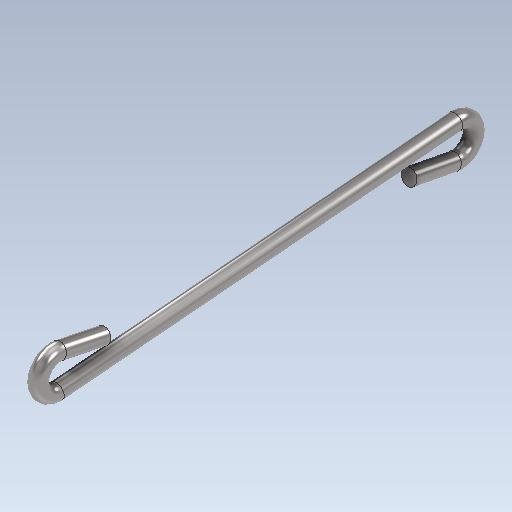
# Autodesk Inventor part: link_4
Saved by Autodesk Inventor 2021 (Build 250183000, 183)
## iProperties
Created: 2023-08-18
Part Number: link_4
Material: Acero inoxidable, 440C
Document SubType Name: Modeling
Designer: Sergio
Density: 7.75 g/cm^3
Appearance: Semipulido
Author: Sergio
Autodesk Inventor part; units mm, degrees
ref_plane "YZ Plane" through (0, 0, 0) normal (1, 0, 0) x (0, 1, 0)
ref_plane "XZ Plane" through (0, 0, 0) normal (0, 1, 0) x (-1, 0, 0)
ref_plane "XY Plane" through (0, 0, 0) normal (0, 0, 1) x (1, 0, 0)
sketch "Boceto1" plane through (0, 0, 0) normal (1, 0, 0) x (0, 1, 0)
  arc A0 (-1.3752, 0.2625) -> (1.3949, 0.119) centre (0, 0) ccw
  line L0 (-1.3949, 59.881) -> (3.6866, 0.3145)
  line L1 (-3.6866, 59.6855) -> (1.3949, 0.119)
  line L2 (-2.5408, 59.7832) -> (2.5408, 0.2168)
  line L3 (0, 53.1) -> (1.3709, 59.7159)
  line L4 (2.2522, 52.6333) -> (3.623, 59.2493)
  line L5 (1.1261, 52.8667) -> (2.497, 59.4826)
  line L6 (-0.1083, 6.8991) -> (-1.3752, 0.2625)
  arc A1 (-2.5048, 0.4781) -> (2.5408, 0.2168) centre (0, 0) ccw
  arc A2 (-3.6344, 0.6937) -> (3.6866, 0.3145) centre (0, 0) ccw
  arc A3 (3.623, 59.2493) -> (-3.6866, 59.6855) centre (0, 60) ccw
  arc A4 (2.497, 59.4826) -> (-2.5408, 59.7832) centre (0, 60) ccw
  arc A5 (1.3709, 59.7159) -> (-1.3949, 59.881) centre (0, 60) ccw
  line L7 (0, 53.1) -> (2.2522, 52.6333)
  line L8 (-0.1083, 6.8991) -> (-2.3675, 7.3304)
  line L9 (-1.2379, 7.1148) -> (-2.5048, 0.4781)
  line L10 (-2.3675, 7.3304) -> (-3.6344, 0.6937)
  dimension "d0" = 2.8
  dimension "d11" = 6.9
  dimension "d12" = 60
  dimension "d13" = 2.3
  dimension "d14" = 1.15
  dimension "d15" = 6.9
  dimension "d22" = 1.4
  dimension "d23" = 0
  dimension "d25" = 1.15
  dimension "d26" = 1.15
  constraints: 22 end point, 12 point on circle, 12 tangent, 6 centre point, 4 parallel, 2 midpoint, 2 perpendicular, 1 coincident
  measures "d0" diameter of A0
  measures "d11" distance of A3.centre L3.start
  measures "d12" distance of A3.centre point (0, 0)
  measures "d13" distance between parallel lines of L3 L4
  measures "d14" distance between parallel lines of L3 L5
  measures "d15" distance of A0.centre L6.start
  measures "d22" radius of A5
  measures "d23" horizontal distance of A3.centre L3.start
  measures "d25" distance between parallel lines of L9 L6
  measures "d26" distance between parallel lines of L10 L9
sketch "Boceto2" plane through (0, 0, 0) normal (0, 1, 0) x (-1, 0, 0)
  line L0 (0, 0) -> (0, -2.55)
  circle A0 centre (0, -2.55) radius 1.15
  dimension "d18" = 2.55
  dimension "d19" = 2.3
  constraints: 2 end point, 1 centre point, 1 coincident, 1 vertical
  measures "d18" distance of L0.start L0.end
  measures "d19" diameter of A0
sweep "Barrido1" add profiles "Boceto2" path "Boceto1" path curves L5 A4 L2 A1 L9
equation "\"d0\" = wire_D + 0.5 * offset"
equation "\"d11\" = 3 * wire_D"
equation "\"d12\" = r4"
equation "\"d13\" = wire_D"
equation "\"d14\" = 0.5 * wire_D"
equation "\"d15\" = 3 * wire_D"
equation "\"d22\" = 0.5 * d0"
equation "\"d25\" = 0.5 * wire_D"
equation "\"d26\" = 0.5 * wire_D"
equation "\"d18\" = 0.5 * d0 + 0.5 * wire_D"
equation "\"d19\" = wire_D"
equation "\"offset\" = 1"
equation "\"r4\" = 60"
equation "\"wire_D\" = 2.3"
equation "\"thikness\" = 2"
equation "\"r1\" = 5.55"
equation "\"r2o\" = 59.75"
equation "\"delta_y\" = 6"
equation "\"wire_d\" = 1"
equation "\"width_ang_spring\" = 5"
equation "\"spring_int_diam\" = 8.5"
equation "\"spring_ext_diam\" = 10.5"
equation "\"r3\" = 8.25"
equation "\"r3R\" = 4.75"
equation "\"r3T\" = 6.74537"
equation "\"alpha\" = 54.847297deg"
equation "\"alpha2\" = 270deg"
equation "\"theta3_recogido\" = 305.152703deg"
equation "\"delta_theta_3\" = 45deg"
equation "\"joint_width\" = 12"
equation "\"joint_radius\" = 7.75"
equation "\"shaft_width\" = 15"
equation "\"shaft_joint_diameter\" = 7.75"
equation "\"separation_space\" = 0.5"
equation "\"height_finger\" = 42"
equation "\"cell_screw_head_diameter\" = 4"
equation "\"cell_screw_diameter\" = 2"
equation "\"cell_space\" = 2"
equation "\"cell_width\" = 6"
equation "\"cell_theta_position\" = 60deg"
equation "\"cell_thikness\" = 1"
equation "\"cell_lenght\" = 37"
equation "\"cell_z_space\" = 5"
equation "\"width_link\" = 8"
equation "\"Dt\" = 1.05949"
equation "\"Djoint_shaft\" = 2.3"
equation "\"shaft_x\" = 1.45"
equation "\"shaft_y\" = 6.45"
equation "\"lenght_body_link\" = 186.05"
equation "\"lenght_bar_support\" = 201.65"
equation "\"trigger_offset\" = 2"
equation "\"m2_theta2o\" = 107deg"
equation "\"m2_r2\" = 28"
equation "\"e\" = 9"
equation "\"So\" = 17"
equation "\"m2_theta3o\" = -30deg"
equation "\"m2_r3\" = 19.75"
equation "\"m2_delta_theta1\" = 15deg"
equation "\"m2_theta3f\" = -60deg"
equation "\"trigger_thumb_lenght\" = 6"
equation "\"width_r12\" = 8"
equation "\"m2_r1\" = 25.2"
equation "\"r3_thikness\" = 3.5"
equation "\"t_thikness\" = 3"
equation "\"tg_width\" = 4"
equation "\"pivot_screw_d\" = 4"
equation "\"pivot_diameter\" = 7"
equation "\"sj_diam_shaft\" = 6"
equation "\"sj_groove\" = 2"
equation "\"sj_groove_deep\" = 7"
equation "\"sj_head_D\" = 7"
equation "\"sj_head_d\" = 4.7464"
equation "\"sj_head_height\" = 5"
equation "\"gj_d\" = 4"
equation "\"gj_out_section\" = 6"
equation "\"sf_head_height\" = 3"
equation "\"screw_lenght\" = 12"
equation "\"screwJ_top_D\" = 13"
equation "\"sf_head_width\" = 4.5"
equation "\"sf_head_grip_width\" = 2"
equation "\"sf_thikness\" = 5"
equation "\"sf_lenght\" = 9.5"
equation "\"sf_head_angle\" = 45deg"
equation "\"sf_base\" = 3"
equation "\"screw_Dhead\" = 8"
equation "\"gj_D\" = 6"
equation "\"screwJ_base_D\" = 9"
equation "\"screw_d\" = 4"
equation "\"sf_head_offset\" = 0.25"
equation "\"spring_lenght\" = 28"
equation "\"spring_int_d\" = 6"
equation "\"wire_spring_d\" = 1"
equation "\"ext_width_slider\" = 3.5"
equation "\"sfbox_tip_width\" = 2.5"
equation "\"slim_width_slider\" = 1.5"
equation "\"agarradera_width\" = 4"
equation "\"int_width_slider\" = 2"
equation "\"agarradera_position\" = 82.13077"
equation "\"sfbox_theta1\" = 60deg"
equation "\"sfbox_theta2\" = 45deg"
equation "\"agarradera_theta\" = 60deg"
equation "\"sfbox_width\" = 1.5"
equation "\"box_fat_slider_lenght\" = 67"
equation "\"fat_width_slider\" = 2"
equation "\"box_in_width\" = 72"
equation "\"flex_separation_theta\" = 60deg"
equation "\"sf_flex_separation\" = 38.66667"
equation "\"thikness_box\" = 1.5"
equation "\"box_slim_slider_lenght\" = 116"
equation "\"box_in_deep\" = 77"
equation "\"box_in_height\" = 35"
